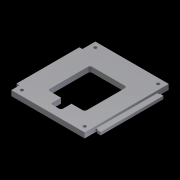
# Autodesk Inventor part: JointA1
Saved by Autodesk Inventor 2011 (Build 150239000, 239)
## iProperties
Created: 2012-10-15
Part Number: JointA1
Document SubType Name: Modeling
Designer: JohnHenry
Density: 1 g/cm^3
Mass: 21.9195 g
Surface Area: 118.837 cm^2
Volume: 21.9195 cm^3
Author: JohnHenry
Autodesk Inventor part; units mm, degrees
ref_plane "YZ Plane" through (0, 0, 0) normal (1, 0, 0) x (0, 1, 0)
ref_plane "XZ Plane" through (0, 0, 0) normal (0, 1, 0) x (-1, 0, 0)
ref_plane "XY Plane" through (0, 0, 0) normal (0, 0, 1) x (1, 0, 0)
sketch "スケッチ1" plane through (0, 0, 0) normal (0, 0, 1) x (1, 0, 0)
  circle A0 centre (0, 0) radius 27.6
  line L0 (-40, 40) -> (40, 40)
  line L1 (40, 40) -> (40, -40)
  line L2 (40, -40) -> (-40, -40)
  line L3 (-40, -40) -> (-40, 40)
  dimension "d0" = 55.2
  dimension "d1" = 40
  dimension "d2" = 80
  dimension "d3" = 80
  dimension "d4" = 40
  constraints: 8 end point, 2 parallel, 1 centre point, 1 coincident, 1 horizontal, 1 perpendicular
  measures "d0" diameter of A0
  measures "d1" distance from line of L0 A0.centre
  measures "d2" distance of L0.end L1.end
  measures "d3" distance of L0.start L0.end
  measures "d4" distance from line of L1 point (0, 0)
extrude "押し出し1" add sketch "スケッチ1" along normal blind 5 contours A0 | L0 L1 L2 L3
sketch "スケッチ3" plane through (0, 0, 5) normal (0, 0, 1) x (1, 0, 0)
  line L0 (40, -40) -> (-40, -40) projected
  line L1 (-40, 40) -> (-34.9, 40)
  line L2 (-34.9, 40) -> (-34.9, -40)
  line L3 (-34.9, -40) -> (-40, -40)
  line L4 (-40, -40) -> (-40, 40)
  line L5 (40, 40) -> (34.9, 40)
  line L6 (34.9, 40) -> (34.9, -40)
  line L7 (34.9, -40) -> (40, -40)
  line L8 (40, -40) -> (40, 40)
  dimension "d17" = 5.1
  dimension "d18" = 5.1
  constraints: 16 end point, 4 parallel, 2 horizontal, 2 perpendicular, 2 point on line
  measures "d17" distance of L2.end L3.end
  measures "d18" distance between parallel lines of L8 L6
extrude "押し出し3" cut sketch "スケッチ3" against normal blind 2.2
sketch "スケッチ4" plane through (0, 0, 0) normal (0, 0, -1) x (-1, 0, 0)
  line L0 (-40, 40) -> (-34.9, 40)
  line L1 (-34.9, 40) -> (-34.9, 29.9)
  line L2 (-34.9, 29.9) -> (-40, 29.9)
  line L3 (-40, 29.9) -> (-40, 40)
  line L4 (-40, -40) -> (-34.9, -40)
  line L5 (-34.9, -40) -> (-34.9, -29.9)
  line L6 (-34.9, -29.9) -> (-40, -29.9)
  line L7 (-40, -29.9) -> (-40, -40)
  line L8 (40, 40) -> (34.9, 40)
  line L9 (34.9, 40) -> (34.9, 29.9)
  line L10 (34.9, 29.9) -> (40, 29.9)
  line L11 (40, 29.9) -> (40, 40)
  line L12 (40, -40) -> (34.9, -40)
  line L13 (34.9, -40) -> (34.9, -29.9)
  line L14 (34.9, -29.9) -> (40, -29.9)
  line L15 (40, -29.9) -> (40, -40)
  dimension "d21" = 5.1
  dimension "d22" = 10.1
  dimension "d23" = 10.1
  dimension "d24" = 10.1
  dimension "d25" = 5.1
  dimension "d26" = 5.1
  dimension "d27" = 5.1
  dimension "d28" = 10.1
  constraints: 32 end point, 8 parallel, 4 horizontal, 4 perpendicular
  measures "d21" distance of L1.end L2.end
  measures "d22" distance of L0.end L1.end
  measures "d23" distance of L4.end L5.end
  measures "d24" distance of L10.end L8.start
  measures "d25" distance of L9.end L10.end
  measures "d26" distance of L5.end L6.end
  measures "d27" distance of L13.end L14.end
  measures "d28" distance of L12.end L13.end
extrude "押し出し4" cut sketch "スケッチ4" against normal through all
sketch "スケッチ5" plane through (0, 0, 0) normal (0, 0, -1) x (-1, 0, 0)
  line L0 (-40, -29.9) -> (-34.9, -29.9) projected
  line L1 (-34.9, -29.9) -> (-34.9, -40) projected
  line L2 (34.9, -40) -> (34.9, -29.9) projected
  line L3 (34.9, -29.9) -> (40, -29.9) projected
  line L4 (40, 29.9) -> (34.9, 29.9) projected
  line L5 (34.9, 29.9) -> (34.9, 40) projected
  line L6 (-34.9, 40) -> (-34.9, 29.9) projected
  line L7 (-34.9, 29.9) -> (-40, 29.9) projected
  point P0 (-35.9, 29.9)
  point P1 (-35.9, -29.9)
  point P2 (35.9, -29.9)
  point P3 (35.9, 29.9)
  dimension "d31" = 1
  dimension "d32" = 1
  dimension "d33" = 1
  dimension "d34" = 1
  constraints: 4 point on line
  measures "d31" distance from line of L6 point (-35.9, 29.9)
  measures "d32" distance from line of L1 point (-35.9, -29.9)
  measures "d33" distance from line of L5 point (35.9, 29.9)
  measures "d34" distance from line of L2 point (35.9, -29.9)
hole "Hole1" at (35.9, 29.9, 0) at (35.9, -29.9, 0) at (-35.9, -29.9, 0) at (-35.9, 29.9, 0) direction (0, 0, 1) diameter 2 end through all
sketch "スケッチ6" plane through (0, 0, 5) normal (0, 0, 1) x (1, 0, 0)
  line L0 (-17.6, 17.6) -> (17.6, 17.6)
  line L1 (17.6, 17.6) -> (17.6, -17.6)
  line L2 (17.6, -17.6) -> (-17.6, -17.6)
  line L3 (-17.6, -17.6) -> (-17.6, 17.6)
  line L4 (-17.6, -17.6) -> (17.6, -17.6)
  line L5 (17.6, -17.6) -> (17.6, -22.6)
  line L6 (17.6, -22.6) -> (-17.6, -22.6)
  line L7 (-17.6, -22.6) -> (-17.6, -17.6)
  point P0 (0, 0)
  dimension "d42" = 35.2
  dimension "d43" = 35.2
  dimension "d44" = 17.6
  dimension "d45" = 17.6
  dimension "d46" = 5
  constraints: 16 end point, 4 parallel, 2 horizontal, 2 perpendicular
  measures "d42" distance of L0.start L0.end
  measures "d43" distance of L0.end L1.end
  measures "d44" distance from line of L1 point (0, 0)
  measures "d45" distance from line of point (0, 0) L0
  measures "d46" distance of L4.end L5.end
extrude "押し出し5" cut sketch "スケッチ6" against normal through all
fillet "フィレット1" radius 2 4 edges at (-17.6, 17.6, 2.5) (-17.6, -22.6, 2.5) (17.6, -22.6, 2.5) (17.6, 17.6, 2.5)
sketch "スケッチ7" plane through (0, 0, 5) normal (0, 0, 1) x (1, 0, 0)
  line L0 (-34.9, 40) -> (-34.9, -40) projected
  line L1 (34.9, -40) -> (-34.9, -40) projected
  line L2 (34.9, -40) -> (34.9, 40) projected
  line L3 (-34.9, 40) -> (34.9, 40) projected
  point P0 (0, 0)
  point P1 (-29.9, 35)
  point P2 (-29.9, -35)
  point P3 (29.9, -35)
  point P4 (29.9, 35)
  dimension "d50" = 5
  dimension "d51" = 5
  dimension "d52" = 5
  dimension "d53" = 5
  dimension "d54" = 5
  dimension "d55" = 5
  dimension "d56" = 5
  dimension "d57" = 5
  measures "d50" distance from line of point (-29.9, 35) L3
  measures "d51" distance from line of L0 point (-29.9, 35)
  measures "d52" distance from line of L2 point (29.9, 35)
  measures "d53" distance from line of L3 point (29.9, 35)
  measures "d54" distance from line of L1 point (-29.9, -35)
  measures "d55" distance from line of L0 point (-29.9, -35)
  measures "d56" distance from line of point (29.9, -35) L2
  measures "d57" distance from line of L1 point (29.9, -35)
hole "Hole2" at (-29.9, 35, 5) at (-29.9, -35, 5) at (29.9, -35, 5) at (29.9, 35, 5) direction (0, 0, -1) diameter 3 end through all
sketch "スケッチ8" plane through (0, 0, 5) normal (0, 0, 1) x (1, 0, 0)
  line L0 (15.6, -22.6) -> (-15.6, -22.6) projected
  line L1 (-5, -22.6) -> (5, -22.6)
  line L2 (5, -22.6) -> (5, -32.6)
  line L3 (5, -32.6) -> (-5, -32.6)
  line L4 (-5, -32.6) -> (-5, -22.6)
  point P0 (0, 0)
  dimension "d65" = 10
  dimension "d66" = 5
  dimension "d67" = 10
  constraints: 8 end point, 2 parallel, 1 horizontal, 1 perpendicular, 1 point on line
  measures "d65" distance of L2.end L3.end
  measures "d66" distance from line of L4 point (0, 0)
  measures "d67" distance of L3.end L1.start
extrude "押し出し6" cut sketch "スケッチ8" against normal through all
fillet "フィレット2" radius 2 2 edges at (-5, -32.6, 2.5) (5, -32.6, 2.5)
equation "\"d1\" = 0.5 * d2"
equation "\"d3\" = d2"
equation "\"d4\" = d1"
equation "\"d18\" = d17"
equation "\"d23\" = d22"
equation "\"d25\" = d21"
equation "\"d26\" = d21"
equation "\"d27\" = d21"
equation "\"d28\" = d22"
equation "\"d32\" = d31"
equation "\"d33\" = d31"
equation "\"d34\" = d31"
equation "\"d44\" = 0.5 * d42"
equation "\"d45\" = d44"
equation "\"d51\" = d50"
equation "\"d52\" = d50"
equation "\"d53\" = d50"
equation "\"d54\" = d50"
equation "\"d55\" = d50"
equation "\"d56\" = d50"
equation "\"d57\" = d50"
equation "\"d66\" = 0.5 * d65"
